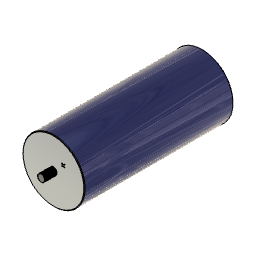
superkondensator (Autodesk Fusion 360 design; units mm, degrees)
Autodesk Fusion 360 part; units mm, degrees
note: some values were not read from the file. Chosen so that the rebuilt part matches the saved one: where a thread starts.
sketch "Szkic1" plane through (0, 0, 0) normal (0, 1, 0) x (1, 0, 0)
  circle A0 centre (0, 0) radius 25
  dimension "d1" = 50
  constraint coincident A0.centre origin
  measures "d1" diameter of A0
extrude "Wyciągnięcie proste1" add sketch "Szkic1" along normal blind 120 makes body 1
sketch "Szkic2" plane through (0, 0, 0) normal (0, -1, 0) x (1, 0, 0)
  circle A0 centre (0, 0) radius 25
  circle A1 centre (0, 0) radius 3
  dimension "d4" = 6
  constraint coincident A0.centre A1.centre
  measures "d4" diameter of A1
extrude "Wyciągnięcie proste2" add sketch "Szkic2" along normal blind 10 contours A1 bodies 1
thread "Gwint1" "ISO Metric profile 6.0 M6x0.5 6g" major diameter 5.927 minor diameter 5.3505 pitch 0.5 angle 60 modelled right hand crest width 0.0685 on face at (2.9963, -6.6667, -0.1495) crest through (2.9635, -9.875, 0) on bodies 1
ref_plane "Płaszczyzna konstrukcyjna1" through (0, 60, 0) normal (0, -1, 0) x (-1, 0, 0)
split "Podział1" by plane through (0, 0, 0) normal (0, -1, 0) bodies 1 makes body 2 at (0.5179, -10, 0.3497)
mirror "Odbij1" about plane through (0, 60, 0) normal (0, -1, 0) of bodies 2 makes body 3
fillet "Zaokrąglenie1" radius 0.5 2 edges at (-23.3082, 120, 9.0404) (-23.3082, 0, 9.0404) on bodies 1
sketch "Szkic3" plane through (0, 0, 0) normal (0, -1, 0) x (1, 0, 0)
  circle A0 centre (0, 0) radius 24.5
  line L0 (-3.1066, 7.5) -> (7.5, -3.1066) construction
  line L1 (7.5, -3.1066) -> (18.1066, 7.5) construction
  line L2 (18.1066, 7.5) -> (7.5, 18.1066) construction
  line L3 (7.5, 18.1066) -> (-3.1066, 7.5) construction
  dimension "d13" = 5
  text T0 "+" font "Arial" height 5 align centre middle in box 15 x 15 at (-3.1066, 7.5) x (0.707107, -0.707107) y (0.707107, 0.707107) spacing 1
extrude "Wyciągnięcie proste3" cut sketch "Szkic3" against normal blind 0.1 text T0 bodies 1
sketch "Szkic4" plane through (0, 120, 0) normal (0, 1, 0) x (-1, 0, 0)
  circle A0 centre (0, 0) radius 24.5
  line L0 (-18.1066, 7.5) -> (-7.5, -3.1066) construction
  line L1 (-7.5, -3.1066) -> (3.1066, 7.5) construction
  line L2 (3.1066, 7.5) -> (-7.5, 18.1066) construction
  line L3 (-7.5, 18.1066) -> (-18.1066, 7.5) construction
  dimension "d16" = 5
  text T0 "-" font "Arial" height 5 align centre middle in box 15 x 15 at (-18.1066, 7.5) x (0.707107, -0.707107) y (0.707107, 0.707107) spacing 1
extrude "Wyciągnięcie proste4" cut sketch "Szkic4" against normal blind 0.1 text T0 bodies 1
